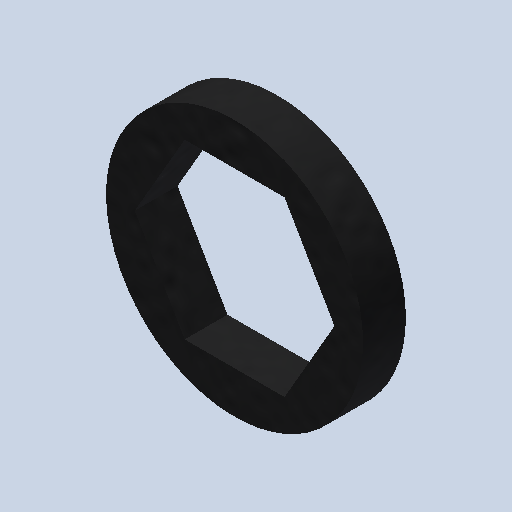
# Autodesk Inventor part: SPACER,HEX,0.125IN
Saved by Autodesk Inventor 2025.2 (Build 292293000, 293)
## iProperties
Category: _
Manager: _
ILogicPurgeVersion: 0.0.0.0
OnSaveVersion: 3.5.0.0
OnSaveAssembly: COREAutomationManager
Created: 2025-03-04
Part Number: SPACER,HEX,0.125IN
Checked By: 00
Engr Approved By: _
User Status: Work In Process
Material: Nylon 6/6
Description: STANDARD (mm)
Document SubType Name: Modeling
Mfg Approved By: John.Thibert
Designer: John.Thibert
Manufacturer: Standard
Standards Organization: Custom
Mass: 0.511377 g
Surface Area: 6.16162 cm^2
Volume: 0.452546 cm^3
Density: 1.13 g/cm^3
Appearance: Black
CN_MASS: 0.0
CN_SERVICEABLE: _
FIRST_DESCRIPTION: _
SECOND_DESCRIPTION: _
THIRD_DESCRIPTION: _
ModelCat: Uncategorized
MaterialName: Nylon 6/6
Subject: _
Author: John.Thibert
Keywords: -
Revision Number: A
Autodesk Inventor part; units mm, degrees
ref_plane "YZ Plane" through (0, 0, 0) normal (1, 0, 0) x (0, 1, 0)
ref_plane "XZ Plane" through (0, 0, 0) normal (0, 1, 0) x (-1, 0, 0)
ref_plane "XY Plane" through (0, 0, 0) normal (0, 0, 1) x (1, 0, 0)
sketch "Sketch2" plane through (0, 0, 0) normal (0, 0, 1) x (1, 0, 0)
  line L0 (-3.7028, -6.4135) -> (-7.4057, 0)
  line L1 (-7.4057, 0) -> (-3.7028, 6.4135)
  line L2 (-3.7028, 6.4135) -> (3.7028, 6.4135)
  line L3 (3.7028, 6.4135) -> (7.4057, 0)
  line L4 (7.4057, 0) -> (3.7028, -6.4135)
  line L5 (3.7028, -6.4135) -> (-3.7028, -6.4135)
  circle A0 centre (0, 0) radius 9.525
  dimension "d0" = 12.827
  dimension "d1" = 19.05
  constraints: 12 end point, 2 coincident, 1 centre point, 1 horizontal, 13 other
  measures "d0" distance between parallel lines of L2 L5
  measures "d1" diameter of A0
extrude "Extrusion1" add sketch "Sketch2" along normal mid plane 3.175
body "Solid1"
